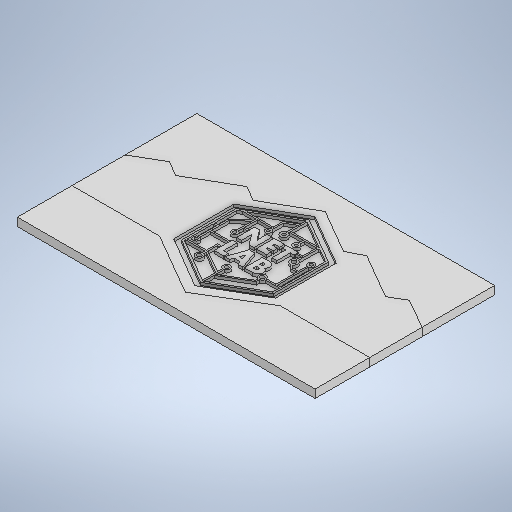
# Autodesk Inventor part: NETLab
Saved by Autodesk Inventor 2025 (Build 290162000, 162)
## iProperties
Created: 2024-07-03
Part Number: NETLab
Material: Generic
Document SubType Name: Modeling
Designer: ethan
Density: 1 g/cm^3
Appearance: Default
Author: ethan
Autodesk Inventor part; units mm, degrees
ref_plane "YZ Plane" through (0, 0, 0) normal (1, 0, 0) x (0, 1, 0)
ref_plane "XZ Plane" through (0, 0, 0) normal (0, 1, 0) x (-1, 0, 0)
ref_plane "XY Plane" through (0, 0, 0) normal (0, 0, 1) x (1, 0, 0)
sketch "Sketch1" plane through (0, 0, 0) normal (0, 1, 0) x (-1, 0, 0)
  line L0 (0, 0) -> (138.1991, 0) construction
  line L1 (138.1991, 0) -> (138.1991, -83.308) construction
  line L2 (138.1991, -83.308) -> (0, -83.308) construction
  line L3 (0, -83.308) -> (0, 0) construction
  line L4 (0, 0) -> (138.1991, 0)
  line L5 (138.1991, 0) -> (138.1991, -83.308)
  line L6 (138.1991, -83.308) -> (0, -83.308)
  line L7 (0, -83.308) -> (0, 0)
  line L8 (0, -57.9492) -> (40.6336, -57.9492)
  line L9 (40.6336, -57.9492) -> (69.1673, -74.5188)
  line L10 (69.1673, -74.5188) -> (96.6084, -57.9492)
  line L11 (96.6084, -57.9492) -> (138.1991, -57.9492)
  line L12 (0, -33.2928) -> (13.016, -25.776)
  line L13 (13.016, -25.776) -> (20.0273, -29.8475)
  line L14 (20.0273, -29.8475) -> (40.9602, -17.7586)
  line L15 (40.9602, -17.7586) -> (47.9764, -21.833)
  line L16 (47.9764, -21.833) -> (69.1673, -9.6112)
  line L17 (69.1673, -9.6112) -> (89.4519, -21.3905)
  line L18 (89.4519, -21.3905) -> (96.6084, -17.7586)
  line L19 (96.6084, -17.7586) -> (117.4261, -29.8475)
  line L20 (117.4261, -29.8475) -> (124.3075, -25.776)
  line L21 (124.3075, -25.776) -> (138.1991, -33.6137)
  line L22 (68.7145, -69.69) -> (92.4856, -55.962)
  line L23 (92.4856, -55.962) -> (92.4856, -27.8088)
  line L24 (92.4856, -27.8088) -> (68.828, -14.0708)
  line L25 (68.828, -14.0708) -> (45.0295, -27.8147)
  line L26 (45.0295, -27.8147) -> (45.0295, -55.7402)
  line L27 (45.0295, -55.7402) -> (68.7145, -69.69)
  line L28 (47.3155, -29.1343) -> (68.8248, -16.7124)
  line L29 (68.8248, -16.7124) -> (90.1996, -29.1248)
  line L30 (90.1996, -29.1248) -> (90.1996, -54.6423)
  line L31 (90.1996, -54.6423) -> (68.7258, -67.0436)
  line L32 (68.7258, -67.0436) -> (47.3155, -54.4335)
  line L33 (47.3155, -54.4335) -> (47.3155, -29.1343)
  line L34 (89.3106, -54.1291) -> (69.058, -65.8252)
  line L35 (68.296, -65.7587) -> (48.2045, -53.9254)
  line L36 (82.219, -25.5185) -> (69.1965, -25.5185)
  line L37 (82.5952, -26.2805) -> (82.5952, -35.3895)
  line L38 (81.8332, -32.6646) -> (79.4067, -32.6646)
  line L39 (79.4067, -32.6646) -> (79.4067, -33.4266)
  line L40 (79.4067, -33.4266) -> (81.8332, -33.4266)
  arc A0 (68.4275, -26.7332) -> (69.1895, -26.7332) centre (68.8085, -28.4048) ccw
  arc A1 (75.6425, -28.3719) -> (76.4045, -28.3719) centre (76.0235, -29.8475) ccw
  circle A2 centre (76.0235, -29.8475) radius 0.635
  circle A3 centre (68.8085, -28.4048) radius 0.8255
  line L41 (87.7165, -35.7087) -> (87.7165, -50.247)
  line L42 (86.9545, -39.8121) -> (84.3196, -39.8121)
  line L43 (84.0628, -40.5741) -> (86.9545, -40.5741)
  circle A4 centre (82.2142, -37.1258) radius 1.016
  line L44 (84.0628, -40.5741) -> (82.4509, -38.8876)
  line L45 (84.3196, -39.8121) -> (83.1791, -38.6188)
  arc A5 (87.7165, -35.7087) -> (86.9545, -35.7087) centre (87.3355, -34.235) ccw
  circle A6 centre (87.3355, -34.235) radius 0.762
  line L46 (80.6251, -53.4443) -> (80.6251, -52.2997)
  circle A7 centre (81.0061, -50.628) radius 0.9525
  line L47 (69.1965, -17.9563) -> (69.1965, -25.5185)
  line L48 (69.1895, -26.2805) -> (69.1895, -26.7332)
  line L49 (69.1895, -26.2805) -> (75.6425, -26.2805)
  line L50 (75.6425, -28.3719) -> (75.6425, -26.2805)
  line L51 (76.4045, -26.2805) -> (76.4045, -28.3719)
  line L52 (76.4045, -26.2805) -> (81.8332, -26.2805)
  line L53 (82.5952, -26.2805) -> (83.5312, -26.2805)
  line L54 (69.1895, -17.9522) -> (82.219, -25.5185)
  line L55 (83.5312, -26.2805) -> (89.3106, -29.6366)
  line L56 (81.8332, -35.3895) -> (81.8332, -33.4266)
  line L57 (81.8332, -32.6646) -> (81.8332, -26.2805)
  arc A8 (81.8332, -35.3895) -> (82.4509, -38.8876) centre (82.2142, -37.1258) ccw
  arc A9 (83.1791, -38.6188) -> (82.5952, -35.3895) centre (82.2142, -37.1258) ccw
  line L58 (86.9545, -50.247) -> (86.9545, -40.5741)
  line L59 (86.9545, -39.8121) -> (86.9545, -35.7087)
  line L60 (89.3106, -50.247) -> (87.7165, -50.247)
  line L61 (86.9545, -50.247) -> (82.6777, -50.247)
  line L62 (82.6708, -51.0075) -> (89.3106, -51.0075)
  line L63 (81.3833, -52.2932) -> (81.3833, -53.827)
  arc A10 (82.6777, -50.247) -> (80.6251, -52.2997) centre (81.0061, -50.628) ccw
  arc A11 (81.3833, -52.2932) -> (82.6708, -51.0075) centre (81.0061, -50.628) ccw
  line L64 (89.3106, -29.6366) -> (89.3106, -50.247)
  line L65 (89.3106, -51.0075) -> (89.3106, -54.1291)
  line L66 (63.404, -23.9384) -> (63.404, -23.4111)
  line L67 (64.166, -23.9384) -> (68.4275, -21.4774)
  line L68 (63.404, -23.4111) -> (68.4275, -20.51)
  line L69 (68.4275, -26.7332) -> (68.4275, -21.4774)
  line L70 (68.4275, -20.51) -> (68.4275, -17.9685)
  line L71 (69.058, -60.2346) -> (80.6251, -53.4443)
  line L72 (69.058, -61.0624) -> (81.3833, -53.827)
  line L73 (48.2045, -52.655) -> (57.1401, -52.655)
  line L74 (57.1401, -53.417) -> (48.2045, -53.417)
  line L75 (48.2045, -53.417) -> (48.2045, -52.655)
  line L76 (57.1401, -47.5851) -> (57.9021, -47.5851)
  line L77 (57.1401, -47.5851) -> (59.0513, -47.5851)
  line L78 (59.0513, -47.5851) -> (59.0513, -48.3471)
  line L79 (59.0513, -48.3471) -> (57.9021, -48.3471)
  line L80 (57.1401, -48.3471) -> (57.1401, -47.5851)
  line L81 (57.9021, -53.5983) -> (68.296, -59.5333)
  line L82 (68.296, -58.7184) -> (57.9021, -52.7835)
  arc A12 (69.058, -56.3744) -> (68.296, -56.3744) centre (68.677, -54.8333) ccw
  circle A13 centre (68.677, -54.8333) radius 0.8255
  arc A14 (57.1401, -54.7407) -> (57.9021, -54.7407) centre (57.5211, -56.4068) ccw
  circle A15 centre (57.5211, -56.4068) radius 0.9525
  line L83 (57.9021, -48.3471) -> (57.9021, -52.7835)
  line L84 (57.9021, -53.5983) -> (57.9021, -54.7407)
  line L85 (57.1401, -54.7407) -> (57.1401, -53.417)
  line L86 (57.1401, -52.655) -> (57.1401, -47.5851)
  line L87 (68.296, -56.3744) -> (68.296, -58.7184)
  line L88 (68.296, -59.5333) -> (68.296, -65.7587)
  line L89 (69.058, -65.7587) -> (69.058, -61.0624)
  line L90 (69.058, -60.2346) -> (69.058, -56.3744)
  line L91 (69.058, -65.7587) -> (69.058, -65.8252)
  arc A16 (63.404, -29.2581) -> (64.166, -29.2581) centre (63.785, -30.6022) ccw
  circle A17 centre (63.785, -30.6022) radius 0.635
  line L92 (51.2065, -27.9138) -> (63.404, -27.9138)
  line L93 (56.8328, -34.6057) -> (59.0513, -34.6057)
  line L94 (59.0513, -34.6057) -> (59.0513, -35.3677)
  line L95 (59.0513, -35.3677) -> (56.8328, -35.3677)
  line L96 (56.8328, -35.3677) -> (56.8328, -35.2468)
  line L97 (48.2045, -39.8121) -> (49.6829, -39.8121)
  line L98 (50.4449, -39.8121) -> (50.4449, -40.5741)
  line L99 (49.6829, -40.5741) -> (48.2045, -40.5741)
  line L100 (50.4449, -43.5538) -> (59.0513, -43.5538)
  line L101 (59.0513, -43.5538) -> (59.0513, -44.3158)
  line L102 (59.0513, -44.3158) -> (50.4449, -44.3158)
  line L103 (49.6829, -39.8121) -> (49.6829, -35.1749)
  line L104 (50.4449, -35.4737) -> (50.4449, -39.8121)
  line L105 (49.6829, -35.1749) -> (56.0708, -29.5993)
  line L106 (50.4449, -35.4737) -> (56.0708, -30.5633)
  arc A18 (56.0708, -37.4772) -> (56.8328, -37.4772) centre (56.4518, -38.8876) ccw
  circle A19 centre (56.4518, -38.8876) radius 0.6985
  line L107 (48.2045, -29.6475) -> (49.887, -28.6758)
  line L108 (51.2065, -27.9138) -> (68.4275, -17.9685)
  line L109 (63.404, -28.6758) -> (56.8328, -28.6758)
  line L110 (56.0708, -28.6758) -> (49.887, -28.6758)
  line L111 (56.0708, -29.5993) -> (56.0708, -28.6758)
  line L112 (64.166, -29.2581) -> (64.166, -23.9384)
  line L113 (56.8328, -28.6758) -> (56.8328, -34.6057)
  line L114 (56.8328, -35.3677) -> (56.8328, -37.4772)
  line L115 (56.0708, -38.3314) -> (56.0708, -38.3022)
  line L116 (56.0708, -37.4772) -> (56.0708, -30.5633)
  line L117 (48.2045, -53.9254) -> (48.2045, -40.5741)
  line L118 (48.2045, -39.8121) -> (48.2045, -29.6475)
  line L119 (50.4449, -43.5538) -> (50.4449, -40.5741)
  line L120 (63.404, -23.9384) -> (63.404, -27.9138)
  line L121 (63.404, -28.6758) -> (63.404, -29.2581)
  line L122 (59.0513, -40.5846) -> (61.3373, -40.5846)
  line L123 (61.3373, -40.5846) -> (61.3373, -35.9047)
  line L124 (61.3373, -32.2425) -> (59.0513, -32.2425)
  line L125 (59.0513, -32.2425) -> (59.0513, -40.5846)
  line L126 (64.8445, -32.2425) -> (67.1305, -32.2425)
  line L127 (67.1305, -32.2425) -> (67.1305, -40.5846)
  line L128 (67.1305, -40.5846) -> (64.8445, -40.5846)
  line L129 (64.8445, -36.9223) -> (64.8445, -32.2425)
  line L130 (64.8445, -40.5846) -> (61.3373, -35.9047)
  line L131 (61.3373, -32.2425) -> (64.8445, -36.9223)
  line L132 (68.1457, -32.2425) -> (70.4317, -32.2425)
  line L133 (70.4317, -40.5846) -> (68.1457, -40.5846)
  line L134 (68.1457, -40.5846) -> (68.1457, -32.2425)
  line L135 (68.1457, -32.2425) -> (72.9255, -32.2425)
  line L136 (72.9255, -32.2425) -> (72.9255, -34.5285)
  line L137 (72.9255, -34.5285) -> (70.4317, -34.5285)
  line L138 (68.1457, -34.5285) -> (68.1457, -32.2425)
  line L139 (70.4317, -35.4304) -> (72.9255, -35.4304)
  line L140 (72.9255, -35.4304) -> (72.9255, -37.4624)
  line L141 (72.9255, -37.4624) -> (70.4317, -37.4624)
  line L142 (68.1457, -37.4624) -> (68.1457, -35.4304)
  line L143 (68.1457, -40.5846) -> (72.9255, -40.5846)
  line L144 (72.9255, -40.5846) -> (72.9255, -38.2986)
  line L145 (72.9255, -38.2986) -> (70.4317, -38.2986)
  line L146 (68.1457, -38.2986) -> (68.1457, -40.5846)
  line L147 (70.4317, -34.5285) -> (70.4317, -35.4304)
  line L148 (70.4317, -37.4624) -> (70.4317, -38.2986)
  line L149 (79.4067, -32.2585) -> (73.7873, -32.2585)
  line L150 (73.7873, -32.2585) -> (73.7873, -34.2905)
  line L151 (79.4067, -34.2905) -> (79.4067, -32.2585)
  line L152 (77.7363, -34.2905) -> (77.7363, -40.5846)
  line L153 (77.7363, -40.5846) -> (75.4503, -40.5846)
  line L154 (75.4503, -40.5846) -> (75.4503, -34.2905)
  line L155 (75.4503, -34.2905) -> (75.6425, -34.2905)
  line L156 (73.7873, -34.2905) -> (75.4503, -34.2905)
  line L157 (77.7363, -34.2905) -> (79.4067, -34.2905)
  line L158 (59.0513, -42.6532) -> (61.3373, -42.6532)
  line L159 (61.3373, -42.6532) -> (61.3373, -48.9755)
  line L160 (61.3373, -51.0075) -> (59.0513, -51.0075)
  line L161 (59.0513, -51.0075) -> (59.0513, -42.6532)
  line L162 (59.0513, -51.0075) -> (63.572, -51.0075)
  line L163 (63.572, -51.0075) -> (63.572, -48.9755)
  line L164 (63.572, -48.9755) -> (61.3373, -48.9755)
  line L165 (59.0513, -48.9755) -> (59.0513, -51.0075)
  line L166 (64.003, -51.0075) -> (66.289, -51.0075)
  line L167 (66.289, -51.0075) -> (66.908, -49.4955)
  line L168 (66.908, -49.4955) -> (69.448, -49.4955)
  line L169 (66.908, -42.6532) -> (69.448, -42.6532)
  line L170 (64.003, -51.0075) -> (66.908, -42.6532)
  line L171 (70.1115, -51.0075) -> (72.3975, -51.0075)
  line L172 (70.1115, -51.0075) -> (69.448, -49.4955)
  line L173 (72.3975, -51.0075) -> (69.448, -42.6532)
  line L174 (67.3012, -47.7499) -> (69.058, -47.7499)
  line L175 (69.058, -47.7499) -> (68.178, -45.6367)
  line L176 (68.178, -45.6367) -> (67.3012, -47.7499)
  line L177 (73.0363, -51.0075) -> (73.0363, -42.6532)
  line L178 (73.0363, -42.6532) -> (76.9663, -42.6532)
  line L179 (73.0363, -51.0075) -> (76.9663, -51.0075)
  line L180 (75.2207, -49.0956) -> (75.2207, -47.596)
  line L181 (75.2207, -45.9499) -> (75.2207, -44.5889)
  line L182 (75.2207, -44.5889) -> (76.0919, -44.5889)
  line L183 (75.2207, -45.9499) -> (76.0919, -45.9499)
  arc A20 (76.0919, -45.9499) -> (76.0919, -44.5889) centre (75.8808, -45.2694) ccw
  line L184 (75.2207, -47.596) -> (76.41, -47.596)
  line L185 (75.2207, -49.0956) -> (76.3936, -49.0956)
  arc A21 (76.3936, -49.0956) -> (76.41, -47.596) centre (76.3353, -48.3451) ccw
  arc A22 (77.8917, -46.4725) -> (76.9663, -42.6532) centre (76.5096, -44.7856) ccw
  arc A23 (76.9663, -51.0075) -> (77.8917, -46.4725) centre (77.088, -48.6704) ccw
  arc A24 (49.6829, -49.0181) -> (50.4449, -49.0181) centre (50.0639, -50.4281) ccw
  circle A25 centre (50.0639, -50.4281) radius 0.6985
  line L186 (49.6829, -40.5741) -> (49.6829, -49.0181)
  line L187 (50.4449, -49.0181) -> (50.4449, -44.3158)
  line L188 (69.1965, -17.9563) -> (82.219, -25.5185)
  line L189 (69.1965, -25.5185) -> (82.219, -25.5185)
  line L190 (69.1965, -25.5185) -> (69.1965, -17.9563)
  constraints: 374 end point, 87 parallel, 37 horizontal, 32 point on circle, 25 centre point, 21 perpendicular, 16 point on line, 10 coincident, 4 collinear, 4 vertical, 15 other
extrude "Extrusion1" add sketch "Sketch1" along normal blind 2.54 contours L4 L5 L21 L20 L19 L18 L17 L16 L15 L14 L13 L12 L7 | L27 L26 L25 L24 L23 L22 | L34 L91 L89 L72 L63 A11 L62 L65 | L35 L117 L74 L85 A14 L84 L81 L88 | L36 L47 L54 | L53 L55 L64 L60 L41 A5 L59 L42 L45 A9 L37 | L38 L151 L149 L150 L156 L154 L153 L152 L157 L40 L56 A8 L44 L43 L58 L61 A10 L46 L71 L90 A12 L87 L82 L83 L79 L161 L160 L162 L163 L164 L159 L158 L100 L119 L98 L104 L106 L116 A18 L114 L95 L125 L122 L123 L130 L128 L127 L126 L129 L131 L124 L93 L113 L109 L121 A16 L112 L67 L69 A0 L48 L49 L50 A1 L51 L52 L57 | L77 L76 L80 L86 L73 L117 L99 L186 A24 L187 L102 L161 | A2 | A3 | A4 | A6 | A7 | L120 L92 L108 L70 L68 L66 | A13 | A15 | A17 | L118 L107 L110 L111 L105 L103 L97 | A19 | L176 L175 L174 | L180 L184 A21 L185 | L181 L182 A20 L183 | A25
sketch "Sketch2" plane through (0, 2.54, 0) normal (0, 1, 0) x (1, 0, 0)
  line L0 (0, 57.9492) -> (-40.6336, 57.9492) projected
  line L1 (-40.6336, 57.9492) -> (-69.1673, 74.5188) projected
  line L2 (-69.1673, 74.5188) -> (-96.6084, 57.9492) projected
  line L3 (-96.6084, 57.9492) -> (-138.1991, 57.9492) projected
  line L4 (-138.1991, 0) -> (-138.1991, 83.308) construction
  line L5 (-138.1991, 83.308) -> (0, 83.308) construction
  line L6 (0, 83.308) -> (0, 0) construction
  line L7 (-138.1991, 57.9492) -> (-138.1991, 83.308)
  line L8 (-138.1991, 83.308) -> (0, 83.308)
  line L9 (0, 83.308) -> (0, 57.9492)
  line L10 (0, 57.9492) -> (-40.6336, 57.9492)
  line L11 (-96.6084, 57.9492) -> (-138.1991, 57.9492)
  constraints: 12 end point, 3 parallel, 2 horizontal, 2 perpendicular
extrude "Extrusion2" add sketch "Sketch2" along normal blind 1.27 and the other way blind 2.54 separate body
sketch "Sketch3" plane through (0, 2.54, 0) normal (0, 1, 0) x (1, 0, 0)
  line L0 (-92.4856, 55.962) -> (-92.4856, 27.8088) projected
  line L1 (-92.4856, 27.8088) -> (-68.828, 14.0708) projected
  line L2 (-68.828, 14.0708) -> (-45.0295, 27.8147) projected
  line L3 (-45.0295, 27.8147) -> (-45.0295, 55.7402) projected
  line L4 (-45.0295, 55.7402) -> (-68.7145, 69.69) projected
  line L5 (-68.7145, 69.69) -> (-92.4856, 55.962) projected
  line L6 (-47.3155, 29.1343) -> (-68.8248, 16.7124) projected
  line L7 (-68.8248, 16.7124) -> (-90.1996, 29.1248) projected
  line L8 (-90.1996, 29.1248) -> (-90.1996, 54.6423) projected
  line L9 (-90.1996, 54.6423) -> (-68.7258, 67.0436) projected
  line L10 (-68.7258, 67.0436) -> (-47.3155, 54.4335) projected
  line L11 (-47.3155, 54.4335) -> (-47.3155, 29.1343) projected
  line L12 (-63.404, 27.9138) -> (-63.404, 23.4111) projected
  line L13 (-63.404, 23.4111) -> (-68.4275, 20.51) projected
  line L14 (-68.4275, 20.51) -> (-68.4275, 17.9685) projected
  line L15 (-68.4275, 17.9685) -> (-51.2065, 27.9138) projected
  line L16 (-51.2065, 27.9138) -> (-63.404, 27.9138) projected
  line L17 (-69.1965, 17.9563) -> (-69.1965, 25.5185) projected
  line L18 (-69.1965, 25.5185) -> (-82.219, 25.5185) projected
  line L19 (-82.219, 25.5185) -> (-69.1965, 17.9563) projected
  line L20 (-81.8332, 26.2805) -> (-76.4045, 26.2805) projected
  line L21 (-76.4045, 26.2805) -> (-76.4045, 28.3719) projected
  arc A0 (-75.6425, 28.3719) -> (-76.4045, 28.3719) centre (-76.0235, 29.8475) ccw projected
  line L22 (-75.6425, 28.3719) -> (-75.6425, 26.2805) projected
  line L23 (-75.6425, 26.2805) -> (-69.1895, 26.2805) projected
  line L24 (-69.1895, 26.2805) -> (-69.1895, 26.7332) projected
  arc A1 (-68.4275, 26.7332) -> (-69.1895, 26.7332) centre (-68.8085, 28.4048) ccw projected
  line L25 (-68.4275, 26.7332) -> (-68.4275, 21.4774) projected
  line L26 (-68.4275, 21.4774) -> (-64.166, 23.9384) projected
  line L27 (-64.166, 23.9384) -> (-64.166, 29.2581) projected
  arc A2 (-63.404, 29.2581) -> (-64.166, 29.2581) centre (-63.785, 30.6022) ccw projected
  line L28 (-63.404, 29.2581) -> (-63.404, 28.6758) projected
  line L29 (-63.404, 28.6758) -> (-56.8328, 28.6758) projected
  line L30 (-56.8328, 28.6758) -> (-56.8328, 34.6057) projected
  line L31 (-56.8328, 34.6057) -> (-59.0513, 34.6057) projected
  line L32 (-59.0513, 34.6057) -> (-59.0513, 32.2425) projected
  line L33 (-59.0513, 32.2425) -> (-61.3373, 32.2425) projected
  line L34 (-61.3373, 32.2425) -> (-64.8445, 36.9223) projected
  line L35 (-64.8445, 36.9223) -> (-64.8445, 32.2425) projected
  line L36 (-64.8445, 32.2425) -> (-67.1305, 32.2425) projected
  line L37 (-67.1305, 32.2425) -> (-67.1305, 40.5846) projected
  line L38 (-67.1305, 40.5846) -> (-64.8445, 40.5846) projected
  line L39 (-64.8445, 40.5846) -> (-61.3373, 35.9047) projected
  line L40 (-61.3373, 35.9047) -> (-61.3373, 40.5846) projected
  line L41 (-61.3373, 40.5846) -> (-59.0513, 40.5846) projected
  line L42 (-59.0513, 40.5846) -> (-59.0513, 35.3677) projected
  line L43 (-59.0513, 35.3677) -> (-56.8328, 35.3677) projected
  line L44 (-56.8328, 35.3677) -> (-56.8328, 37.4772) projected
  arc A3 (-56.0708, 37.4772) -> (-56.8328, 37.4772) centre (-56.4518, 38.8876) ccw projected
  line L45 (-56.0708, 37.4772) -> (-56.0708, 30.5633) projected
  line L46 (-56.0708, 30.5633) -> (-50.4449, 35.4737) projected
  line L47 (-50.4449, 35.4737) -> (-50.4449, 43.5538) projected
  line L48 (-50.4449, 43.5538) -> (-59.0513, 43.5538) projected
  line L49 (-59.0513, 43.5538) -> (-59.0513, 42.6532) projected
  line L50 (-59.0513, 42.6532) -> (-61.3373, 42.6532) projected
  line L51 (-61.3373, 42.6532) -> (-61.3373, 48.9755) projected
  line L52 (-61.3373, 48.9755) -> (-63.572, 48.9755) projected
  line L53 (-63.572, 48.9755) -> (-63.572, 51.0075) projected
  line L54 (-63.572, 51.0075) -> (-59.0513, 51.0075) projected
  line L55 (-59.0513, 51.0075) -> (-59.0513, 48.3471) projected
  line L56 (-59.0513, 48.3471) -> (-57.9021, 48.3471) projected
  line L57 (-57.9021, 48.3471) -> (-57.9021, 52.7835) projected
  line L58 (-57.9021, 52.7835) -> (-68.296, 58.7184) projected
  line L59 (-68.296, 58.7184) -> (-68.296, 56.3744) projected
  arc A4 (-69.058, 56.3744) -> (-68.296, 56.3744) centre (-68.677, 54.8333) ccw projected
  line L60 (-69.058, 56.3744) -> (-69.058, 60.2346) projected
  line L61 (-69.058, 60.2346) -> (-80.6251, 53.4443) projected
  line L62 (-80.6251, 53.4443) -> (-80.6251, 52.2997) projected
  arc A5 (-82.6777, 50.247) -> (-80.6251, 52.2997) centre (-81.0061, 50.628) ccw projected
  line L63 (-82.6777, 50.247) -> (-86.9545, 50.247) projected
  line L64 (-86.9545, 50.247) -> (-86.9545, 40.5741) projected
  line L65 (-86.9545, 40.5741) -> (-84.0628, 40.5741) projected
  line L66 (-84.0628, 40.5741) -> (-82.4509, 38.8876) projected
  arc A6 (-81.8332, 35.3895) -> (-82.4509, 38.8876) centre (-82.2142, 37.1258) ccw projected
  line L67 (-81.8332, 35.3895) -> (-81.8332, 33.4266) projected
  line L68 (-81.8332, 33.4266) -> (-79.4067, 33.4266) projected
  line L69 (-79.4067, 33.4266) -> (-79.4067, 34.2905) projected
  line L70 (-79.4067, 34.2905) -> (-77.7363, 34.2905) projected
  line L71 (-77.7363, 34.2905) -> (-77.7363, 40.5846) projected
  line L72 (-77.7363, 40.5846) -> (-75.4503, 40.5846) projected
  line L73 (-75.4503, 40.5846) -> (-75.4503, 34.2905) projected
  line L74 (-75.4503, 34.2905) -> (-73.7873, 34.2905) projected
  line L75 (-73.7873, 34.2905) -> (-73.7873, 32.2585) projected
  line L76 (-73.7873, 32.2585) -> (-79.4067, 32.2585) projected
  line L77 (-79.4067, 32.2585) -> (-79.4067, 32.6646) projected
  line L78 (-79.4067, 32.6646) -> (-81.8332, 32.6646) projected
  line L79 (-81.8332, 32.6646) -> (-81.8332, 26.2805) projected
  line L80 (-72.9255, 32.2425) -> (-72.9255, 34.5285) projected
  line L81 (-72.9255, 34.5285) -> (-70.4317, 34.5285) projected
  line L82 (-70.4317, 34.5285) -> (-70.4317, 35.4304) projected
  line L83 (-70.4317, 35.4304) -> (-72.9255, 35.4304) projected
  line L84 (-72.9255, 35.4304) -> (-72.9255, 37.4624) projected
  line L85 (-72.9255, 37.4624) -> (-70.4317, 37.4624) projected
  line L86 (-70.4317, 37.4624) -> (-70.4317, 38.2986) projected
  line L87 (-70.4317, 38.2986) -> (-72.9255, 38.2986) projected
  line L88 (-72.9255, 38.2986) -> (-72.9255, 40.5846) projected
  line L89 (-72.9255, 40.5846) -> (-68.1457, 40.5846) projected
  line L90 (-68.1457, 40.5846) -> (-68.1457, 32.2425) projected
  line L91 (-68.1457, 32.2425) -> (-72.9255, 32.2425) projected
  line L92 (-76.9663, 51.0075) -> (-73.0363, 51.0075) projected
  line L93 (-73.0363, 51.0075) -> (-73.0363, 42.6532) projected
  line L94 (-73.0363, 42.6532) -> (-76.9663, 42.6532) projected
  arc A7 (-77.8917, 46.4725) -> (-76.9663, 42.6532) centre (-76.5096, 44.7856) ccw projected
  arc A8 (-76.9663, 51.0075) -> (-77.8917, 46.4725) centre (-77.088, 48.6704) ccw projected
  line L95 (-66.908, 42.6532) -> (-69.448, 42.6532) projected
  line L96 (-69.448, 42.6532) -> (-72.3975, 51.0075) projected
  line L97 (-72.3975, 51.0075) -> (-70.1115, 51.0075) projected
  line L98 (-70.1115, 51.0075) -> (-69.448, 49.4955) projected
  line L99 (-69.448, 49.4955) -> (-66.908, 49.4955) projected
  line L100 (-66.908, 49.4955) -> (-66.289, 51.0075) projected
  line L101 (-66.289, 51.0075) -> (-64.003, 51.0075) projected
  line L102 (-64.003, 51.0075) -> (-66.908, 42.6532) projected
  line L103 (-82.5952, 26.2805) -> (-82.5952, 35.3895) projected
  arc A9 (-83.1791, 38.6188) -> (-82.5952, 35.3895) centre (-82.2142, 37.1258) ccw projected
  line L104 (-83.1791, 38.6188) -> (-84.3196, 39.8121) projected
  line L105 (-84.3196, 39.8121) -> (-86.9545, 39.8121) projected
  line L106 (-86.9545, 39.8121) -> (-86.9545, 35.7087) projected
  arc A10 (-87.7165, 35.7087) -> (-86.9545, 35.7087) centre (-87.3355, 34.235) ccw projected
  line L107 (-87.7165, 35.7087) -> (-87.7165, 50.247) projected
  line L108 (-87.7165, 50.247) -> (-89.3106, 50.247) projected
  line L109 (-89.3106, 50.247) -> (-89.3106, 29.6366) projected
  line L110 (-89.3106, 29.6366) -> (-83.5312, 26.2805) projected
  line L111 (-83.5312, 26.2805) -> (-82.5952, 26.2805) projected
  line L112 (-81.3833, 53.827) -> (-69.058, 61.0624) projected
  line L113 (-69.058, 61.0624) -> (-69.058, 65.8252) projected
  line L114 (-69.058, 65.8252) -> (-89.3106, 54.1291) projected
  line L115 (-89.3106, 54.1291) -> (-89.3106, 51.0075) projected
  line L116 (-89.3106, 51.0075) -> (-82.6708, 51.0075) projected
  arc A11 (-81.3833, 52.2932) -> (-82.6708, 51.0075) centre (-81.0061, 50.628) ccw projected
  line L117 (-81.3833, 52.2932) -> (-81.3833, 53.827) projected
  line L118 (-68.296, 65.7587) -> (-68.296, 59.5333) projected
  line L119 (-68.296, 59.5333) -> (-57.9021, 53.5983) projected
  line L120 (-57.9021, 53.5983) -> (-57.9021, 54.7407) projected
  arc A12 (-57.1401, 54.7407) -> (-57.9021, 54.7407) centre (-57.5211, 56.4068) ccw projected
  line L121 (-57.1401, 54.7407) -> (-57.1401, 53.417) projected
  line L122 (-57.1401, 53.417) -> (-48.2045, 53.417) projected
  line L123 (-48.2045, 53.417) -> (-48.2045, 53.9254) projected
  line L124 (-48.2045, 53.9254) -> (-68.296, 65.7587) projected
  arc A13 (-49.6829, 49.0181) -> (-50.4449, 49.0181) centre (-50.0639, 50.4281) ccw projected
  line L125 (-49.6829, 49.0181) -> (-49.6829, 40.5741) projected
  line L126 (-49.6829, 40.5741) -> (-48.2045, 40.5741) projected
  line L127 (-48.2045, 40.5741) -> (-48.2045, 52.655) projected
  line L128 (-48.2045, 52.655) -> (-57.1401, 52.655) projected
  line L129 (-57.1401, 52.655) -> (-57.1401, 47.5851) projected
  line L130 (-57.1401, 47.5851) -> (-59.0513, 47.5851) projected
  line L131 (-59.0513, 47.5851) -> (-59.0513, 44.3158) projected
  line L132 (-59.0513, 44.3158) -> (-50.4449, 44.3158) projected
  line L133 (-50.4449, 44.3158) -> (-50.4449, 49.0181) projected
  line L134 (-48.2045, 39.8121) -> (-49.6829, 39.8121) projected
  line L135 (-49.6829, 39.8121) -> (-49.6829, 35.1749) projected
  line L136 (-49.6829, 35.1749) -> (-56.0708, 29.5993) projected
  line L137 (-56.0708, 29.5993) -> (-56.0708, 28.6758) projected
  line L138 (-56.0708, 28.6758) -> (-49.887, 28.6758) projected
  line L139 (-49.887, 28.6758) -> (-48.2045, 29.6475) projected
  line L140 (-48.2045, 29.6475) -> (-48.2045, 39.8121) projected
  line L141 (-59.0513, 34.6057) -> (-59.0513, 32.2425) projected
  line L142 (-59.0513, 35.3677) -> (-59.0513, 34.6057)
  line L143 (-79.4067, 33.4266) -> (-79.4067, 32.6646)
  line L144 (-81.8332, 33.4266) -> (-79.4067, 33.4266) projected
  line L145 (-59.0513, 44.3158) -> (-59.0513, 43.5538)
  line L146 (-59.0513, 48.3471) -> (-59.0513, 47.5851)
  circle A14 centre (-63.785, 30.6022) radius 0.635 projected
  circle A15 centre (-68.8085, 28.4048) radius 0.8255 projected
  circle A16 centre (-76.0235, 29.8475) radius 0.635 projected
  circle A17 centre (-82.2142, 37.1258) radius 1.016 projected
  circle A18 centre (-87.3355, 34.235) radius 0.762 projected
  circle A19 centre (-81.0061, 50.628) radius 0.9525 projected
  circle A20 centre (-68.677, 54.8333) radius 0.8255 projected
  circle A21 centre (-57.5211, 56.4068) radius 0.9525 projected
  circle A22 centre (-50.0639, 50.4281) radius 0.6985 projected
  circle A23 centre (-56.4518, 38.8876) radius 0.6985 projected
  point P0 (0, 0)
  constraints: 8 end point, 2 collinear, 1 perpendicular, 1 vertical
extrude "Extrusion3" add sketch "Sketch3" along normal blind 1.27 and the other way blind 2.54 separate body contours L6 L7 L8 L9 L10 L11
sketch "Sketch4" plane through (0, 2.54, 0) normal (0, 1, 0) x (1, 0, 0)
  line L0 (0, 0) -> (0, 33.2928)
  line L1 (0, 33.2928) -> (-13.016, 25.776)
  line L2 (-13.016, 25.776) -> (-20.0273, 29.8475)
  line L3 (-20.0273, 29.8475) -> (-40.9602, 17.7586)
  line L4 (-40.9602, 17.7586) -> (-47.9764, 21.833)
  line L5 (-47.9764, 21.833) -> (-69.1673, 9.6112)
  line L6 (-69.1673, 9.6112) -> (-89.4519, 21.3905)
  line L7 (-89.4519, 21.3905) -> (-96.6084, 17.7586)
  line L8 (-96.6084, 17.7586) -> (-117.4261, 29.8475)
  line L9 (-117.4261, 29.8475) -> (-124.3075, 25.776)
  line L10 (-124.3075, 25.776) -> (-138.1991, 33.6137)
  line L11 (-138.1991, 33.6137) -> (-138.1991, 0)
  line L12 (-138.1991, 0) -> (0, 0)
  line L13 (-69.1673, 74.5188) -> (-40.6336, 57.9492)
  line L14 (-40.6336, 57.9492) -> (0, 57.9492)
  line L15 (0, 57.9492) -> (0, 83.308)
  line L16 (0, 83.308) -> (-138.1991, 83.308)
  line L17 (-138.1991, 83.308) -> (-138.1991, 57.9492)
  line L18 (-138.1991, 57.9492) -> (-96.6084, 57.9492)
  line L19 (-96.6084, 57.9492) -> (-69.1673, 74.5188)
  line L20 (-92.4856, 55.962) -> (-92.4856, 27.8088)
  line L21 (-92.4856, 27.8088) -> (-68.828, 14.0708)
  line L22 (-68.828, 14.0708) -> (-45.0295, 27.8147)
  line L23 (-45.0295, 27.8147) -> (-45.0295, 55.7402)
  line L24 (-45.0295, 55.7402) -> (-68.7145, 69.69)
  line L25 (-68.7145, 69.69) -> (-92.4856, 55.962)
  line L26 (-47.3155, 29.1343) -> (-68.8248, 16.7124)
  line L27 (-68.8248, 16.7124) -> (-90.1996, 29.1248)
  line L28 (-90.1996, 29.1248) -> (-90.1996, 54.6423)
  line L29 (-90.1996, 54.6423) -> (-68.7258, 67.0436)
  line L30 (-68.7258, 67.0436) -> (-47.3155, 54.4335)
  line L31 (-47.3155, 54.4335) -> (-47.3155, 29.1343)
  line L32 (0, 57.9492) -> (0, 33.2928)
  line L33 (-138.1991, 57.9492) -> (-96.6084, 57.9492)
  line L34 (-138.1991, 57.9492) -> (-138.1991, 33.6137)
  line L35 (-81.8332, 26.2805) -> (-76.4045, 26.2805)
  line L36 (-76.4045, 26.2805) -> (-76.4045, 28.3719)
  arc A0 (-75.6425, 28.3719) -> (-76.4045, 28.3719) centre (-76.0235, 29.8475) ccw
  line L37 (-75.6425, 28.3719) -> (-75.6425, 26.2805)
  line L38 (-75.6425, 26.2805) -> (-69.1895, 26.2805)
  line L39 (-69.1895, 26.2805) -> (-69.1895, 26.7332)
  arc A1 (-68.4275, 26.7332) -> (-69.1895, 26.7332) centre (-68.8085, 28.4048) ccw
  line L40 (-68.4275, 26.7332) -> (-68.4275, 21.4774)
  line L41 (-68.4275, 21.4774) -> (-64.166, 23.9384)
  line L42 (-64.166, 23.9384) -> (-64.166, 29.2581)
  arc A2 (-63.404, 29.2581) -> (-64.166, 29.2581) centre (-63.785, 30.6022) ccw
  line L43 (-63.404, 29.2581) -> (-63.404, 28.6758)
  line L44 (-63.404, 28.6758) -> (-56.8328, 28.6758)
  line L45 (-56.8328, 28.6758) -> (-56.8328, 34.6057)
  line L46 (-56.8328, 34.6057) -> (-59.0513, 34.6057)
  line L47 (-59.0513, 34.6057) -> (-59.0513, 32.2425)
  line L48 (-59.0513, 32.2425) -> (-61.3373, 32.2425)
  line L49 (-61.3373, 32.2425) -> (-64.8445, 36.9223)
  line L50 (-64.8445, 36.9223) -> (-64.8445, 32.2425)
  line L51 (-64.8445, 32.2425) -> (-67.1305, 32.2425)
  line L52 (-67.1305, 32.2425) -> (-67.1305, 40.5846)
  line L53 (-67.1305, 40.5846) -> (-64.8445, 40.5846)
  line L54 (-64.8445, 40.5846) -> (-61.3373, 35.9047)
  line L55 (-61.3373, 35.9047) -> (-61.3373, 40.5846)
  line L56 (-61.3373, 40.5846) -> (-59.0513, 40.5846)
  line L57 (-59.0513, 40.5846) -> (-59.0513, 35.3677)
  line L58 (-59.0513, 35.3677) -> (-56.8328, 35.3677)
  line L59 (-56.8328, 35.3677) -> (-56.8328, 37.4772)
  arc A3 (-56.0708, 37.4772) -> (-56.8328, 37.4772) centre (-56.4518, 38.8876) ccw
  line L60 (-56.0708, 37.4772) -> (-56.0708, 30.5633)
  line L61 (-56.0708, 30.5633) -> (-50.4449, 35.4737)
  line L62 (-50.4449, 35.4737) -> (-50.4449, 43.5538)
  line L63 (-50.4449, 43.5538) -> (-59.0513, 43.5538)
  line L64 (-59.0513, 43.5538) -> (-59.0513, 42.6532)
  line L65 (-59.0513, 42.6532) -> (-61.3373, 42.6532)
  line L66 (-61.3373, 42.6532) -> (-61.3373, 48.9755)
  line L67 (-61.3373, 48.9755) -> (-63.572, 48.9755)
  line L68 (-63.572, 48.9755) -> (-63.572, 51.0075)
  line L69 (-63.572, 51.0075) -> (-59.0513, 51.0075)
  line L70 (-59.0513, 51.0075) -> (-59.0513, 48.3471)
  line L71 (-59.0513, 48.3471) -> (-57.9021, 48.3471)
  line L72 (-57.9021, 48.3471) -> (-57.9021, 52.7835)
  line L73 (-57.9021, 52.7835) -> (-68.296, 58.7184)
  line L74 (-68.296, 58.7184) -> (-68.296, 56.3744)
  arc A4 (-69.058, 56.3744) -> (-68.296, 56.3744) centre (-68.677, 54.8333) ccw
  line L75 (-69.058, 56.3744) -> (-69.058, 60.2346)
  line L76 (-69.058, 60.2346) -> (-80.6251, 53.4443)
  line L77 (-80.6251, 53.4443) -> (-80.6251, 52.2997)
  arc A5 (-82.6777, 50.247) -> (-80.6251, 52.2997) centre (-81.0061, 50.628) ccw
  line L78 (-82.6777, 50.247) -> (-86.9545, 50.247)
  line L79 (-86.9545, 50.247) -> (-86.9545, 40.5741)
  line L80 (-86.9545, 40.5741) -> (-84.0628, 40.5741)
  line L81 (-84.0628, 40.5741) -> (-82.4509, 38.8876)
  arc A6 (-81.8332, 35.3895) -> (-82.4509, 38.8876) centre (-82.2142, 37.1258) ccw
  line L82 (-81.8332, 35.3895) -> (-81.8332, 33.4266)
  line L83 (-81.8332, 33.4266) -> (-79.4067, 33.4266)
  line L84 (-79.4067, 33.4266) -> (-79.4067, 34.2905)
  line L85 (-79.4067, 34.2905) -> (-77.7363, 34.2905)
  line L86 (-77.7363, 34.2905) -> (-77.7363, 40.5846)
  line L87 (-77.7363, 40.5846) -> (-75.4503, 40.5846)
  line L88 (-75.4503, 40.5846) -> (-75.4503, 34.2905)
  line L89 (-75.4503, 34.2905) -> (-73.7873, 34.2905)
  line L90 (-73.7873, 34.2905) -> (-73.7873, 32.2585)
  line L91 (-73.7873, 32.2585) -> (-79.4067, 32.2585)
  line L92 (-79.4067, 32.2585) -> (-79.4067, 32.6646)
  line L93 (-79.4067, 32.6646) -> (-81.8332, 32.6646)
  line L94 (-81.8332, 32.6646) -> (-81.8332, 26.2805)
  line L95 (-72.9255, 32.2425) -> (-72.9255, 34.5285)
  line L96 (-72.9255, 34.5285) -> (-70.4317, 34.5285)
  line L97 (-70.4317, 34.5285) -> (-70.4317, 35.4304)
  line L98 (-70.4317, 35.4304) -> (-72.9255, 35.4304)
  line L99 (-72.9255, 35.4304) -> (-72.9255, 37.4624)
  line L100 (-72.9255, 37.4624) -> (-70.4317, 37.4624)
  line L101 (-70.4317, 37.4624) -> (-70.4317, 38.2986)
  line L102 (-70.4317, 38.2986) -> (-72.9255, 38.2986)
  line L103 (-72.9255, 38.2986) -> (-72.9255, 40.5846)
  line L104 (-72.9255, 40.5846) -> (-68.1457, 40.5846)
  line L105 (-68.1457, 40.5846) -> (-68.1457, 32.2425)
  line L106 (-68.1457, 32.2425) -> (-72.9255, 32.2425)
  line L107 (-76.9663, 51.0075) -> (-73.0363, 51.0075)
  line L108 (-73.0363, 51.0075) -> (-73.0363, 42.6532)
  line L109 (-73.0363, 42.6532) -> (-76.9663, 42.6532)
  arc A7 (-77.8917, 46.4725) -> (-76.9663, 42.6532) centre (-76.5096, 44.7856) ccw
  arc A8 (-76.9663, 51.0075) -> (-77.8917, 46.4725) centre (-77.088, 48.6704) ccw
  line L110 (-66.908, 42.6532) -> (-69.448, 42.6532)
  line L111 (-69.448, 42.6532) -> (-72.3975, 51.0075)
  line L112 (-72.3975, 51.0075) -> (-70.1115, 51.0075)
  line L113 (-70.1115, 51.0075) -> (-69.448, 49.4955)
  line L114 (-69.448, 49.4955) -> (-66.908, 49.4955)
  line L115 (-66.908, 49.4955) -> (-66.289, 51.0075)
  line L116 (-66.289, 51.0075) -> (-64.003, 51.0075)
  line L117 (-64.003, 51.0075) -> (-66.908, 42.6532)
  line L118 (-59.0513, 40.5846) -> (-59.0513, 35.3677)
  line L119 (-59.0513, 35.3677) -> (-59.0513, 34.6057)
  line L120 (-79.4067, 33.4266) -> (-79.4067, 32.6646)
  line L121 (-59.0513, 47.5851) -> (-59.0513, 44.3158)
  line L122 (-59.0513, 48.3471) -> (-59.0513, 47.5851)
  line L123 (-59.0513, 47.5851) -> (-59.0513, 44.3158)
  line L124 (-59.0513, 44.3158) -> (-59.0513, 43.5538)
  line L125 (-76.0919, 44.5889) -> (-75.2207, 44.5889)
  line L126 (-75.2207, 44.5889) -> (-75.2207, 45.9499)
  line L127 (-75.2207, 45.9499) -> (-76.0919, 45.9499)
  arc A9 (-76.0919, 45.9499) -> (-76.0919, 44.5889) centre (-75.8808, 45.2694) ccw
  line L128 (-76.41, 47.596) -> (-75.2207, 47.596)
  line L129 (-75.2207, 47.596) -> (-75.2207, 49.0956)
  line L130 (-75.2207, 49.0956) -> (-76.3936, 49.0956)
  arc A10 (-76.3936, 49.0956) -> (-76.41, 47.596) centre (-76.3353, 48.3451) ccw
  line L131 (-69.058, 47.7499) -> (-68.178, 45.6367)
  line L132 (-68.178, 45.6367) -> (-67.3012, 47.7499)
  line L133 (-67.3012, 47.7499) -> (-69.058, 47.7499)
extrude "Extrusion4" add sketch "Sketch4" along normal blind 1.27 and the other way blind 2.54 separate body contours L1 L2 L3 L4 L5 L6 L7 L8 L9 L10 L34 L18 L19 L13 L14 L32 | L120 L84 L85 L86 L87 L88 L89 L90 L91 L92 | L47 L48 L49 L50 L51 L52 L53 L54 L55 L56 L57 L119 | L122 L121 L124 L64 L65 L66 L67 L68 L69 L70 | L95 L96 L97 L98 L99 L100 L101 L102 L103 L104 L105 L106 | L107 L108 L109 A7 A8 | L110 L111 L112 L113 L114 L115 L116 L117
sketch "Sketch5" plane through (0, 2.54, 0) normal (0, 1, 0) x (1, 0, 0)
  line L0 (0, 0) -> (0, 33.2928) projected
  line L1 (0, 33.2928) -> (-13.016, 25.776) projected
  line L2 (-13.016, 25.776) -> (-20.0273, 29.8475) projected
  line L3 (-20.0273, 29.8475) -> (-40.9602, 17.7586) projected
  line L4 (-40.9602, 17.7586) -> (-47.9764, 21.833) projected
  line L5 (-47.9764, 21.833) -> (-69.1673, 9.6112) projected
  line L6 (-69.1673, 9.6112) -> (-89.4519, 21.3905) projected
  line L7 (-89.4519, 21.3905) -> (-96.6084, 17.7586) projected
  line L8 (-96.6084, 17.7586) -> (-117.4261, 29.8475) projected
  line L9 (-117.4261, 29.8475) -> (-124.3075, 25.776) projected
  line L10 (-124.3075, 25.776) -> (-138.1991, 33.6137) projected
  line L11 (-138.1991, 33.6137) -> (-138.1991, 0) projected
  line L12 (-138.1991, 0) -> (0, 0) projected
extrude "Extrusion5" add sketch "Sketch5" along normal blind 1.27 bodies 1
body "Solid1"
body "Solid2"
body "Solid3"
body "Solid4"
